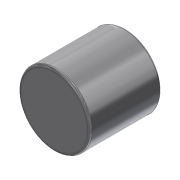
# Autodesk Inventor part: Part6
Saved by Autodesk Inventor 2014 (Build 180170000, 170)
## iProperties
Created: 2016-03-03
Part Number: Part6
Material: Silver
Document SubType Name: Modeling
Designer: admin
Density: 10.49 g/cm^3
Appearance: Silver
Author: admin
Autodesk Inventor part; units mm, degrees
ref_plane "YZ Plane" through (0, 0, 0) normal (1, 0, 0) x (0, 1, 0)
ref_plane "XZ Plane" through (0, 0, 0) normal (0, 1, 0) x (-1, 0, 0)
ref_plane "XY Plane" through (0, 0, 0) normal (0, 0, 1) x (1, 0, 0)
sketch "Sketch1" plane through (0, 0, 0) normal (0, 1, 0) x (-1, 0, 0)
  circle A0 centre (0, 0) radius 5
  dimension "d0" = 10
  constraints: 1 centre point, 1 coincident
  measures "d0" diameter of A0
extrude "Extrusion1" add sketch "Sketch1" along normal blind 10
fillet "Fillet1" radius 0.3 2 edges at (5, 10, 0) (5, 0, 0)
body "Solid1"
